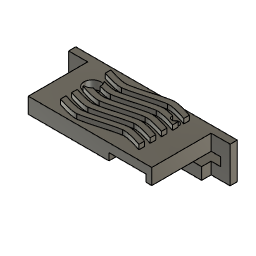
Enviro Module Cover Plate (Autodesk Fusion 360 design; units mm, degrees)
Autodesk Fusion 360 part; units mm, degrees
sketch "Sketch1" plane through (0, 0, 0) normal (0, 0, 1) x (1, 0, 0)
  line L0 (0, 0) -> (26, 0)
  line L1 (26, 0) -> (26, 16)
  line L2 (26, 16) -> (0, 16)
  line L3 (0, 16) -> (0, 0)
  dimension "d1" = 26
  dimension "d2" = 16
  constraint horizontal L0
  constraint vertical L1
  constraint horizontal L2
  constraint vertical L3
  constraint coincident L0.start L3.end
  measures "d1" horizontal distance of L0.start L0.end
  measures "d2" vertical distance of L0.start L2.end
extrude "Extrude1" add sketch "Sketch1" along normal blind 3.3
sketch "Sketch2" plane through (0, 0, 0) normal (0, 0, 1) x (1, 0, 0)
  line L0 (0, 16) -> (26, 16)
  line L1 (26, 16) -> (26, 14.5)
  line L2 (26, 14.5) -> (0, 14.5)
  line L3 (0, 14.5) -> (0, 16)
  point P0 (0, 16)
  dimension "d5" = 1.5
  constraint horizontal L0
  constraint vertical L1
  constraint horizontal L2
  constraint vertical L3
  constraint coincident P0 L0.start
  measures "d5" vertical distance of P0 L2.end
extrude "Extrude2" add sketch "Sketch2" against normal blind 1.8
sketch "Sketch3" plane through (0, 0, 0) normal (0, 0, -1) x (1, 0, 0)
  line L0 (0, -14.5) -> (26, -14.5)
  line L1 (26, -14.5) -> (26, 0)
  line L2 (26, 0) -> (0, 0)
  line L3 (0, 0) -> (0, -14.5)
  line L4 (0, -10) -> (2, -10)
  line L5 (2, -10) -> (2, -4.5)
  line L6 (2, -4.5) -> (17, -4.5)
  line L7 (17, -4.5) -> (17, 0)
  line L8 (17, 0) -> (24.8, 0)
  line L9 (24.8, 0) -> (24.8, -14.5)
  line L10 (0, -11.5) -> (2, -11.5)
  line L11 (2, -11.5) -> (2, -14.5)
  dimension "d8" = 1.2
  dimension "d9" = 14.5
  dimension "d10" = 10
  dimension "d11" = 2
  dimension "d12" = 3
  dimension "d13" = 1.5
  dimension "d14" = 9
  constraint perpendicular L3 L4
  constraint perpendicular L4 L5
  constraint perpendicular L5 L6
  constraint perpendicular L6 L7
  constraint perpendicular L5 L8
  constraint perpendicular L0 L9
  constraint coincident L0 L9.end
  constraint coincident L3 L4.start
  constraint coincident L3 L10.start
  constraint perpendicular L3 L10
  constraint coincident L0 L11.end
  constraint perpendicular L0 L11
  constraint collinear L5 L11
  measures "d8" distance of L1 L9
  measures "d9" distance of L8 L9.end
  measures "d10" distance of L0 L6
  measures "d11" distance of L3 L11
  measures "d12" distance of L0 L10
  measures "d13" distance of L4 L10
  measures "d14" distance of L1 L7
extrude "Extrude3" cut sketch "Sketch3" against normal blind 1.5 contours L0 L2 L3 L4 L5 L6 L7 L8 L9 L10 L11
sketch "Sketch4" plane through (0, 0, -1.8) normal (0, 0, -1) x (1, 0, 0)
  line L0 (26, -14.5) -> (0, -14.5)
  line L1 (0, -14.5) -> (0, -16)
  line L2 (0, -16) -> (26, -16)
  line L3 (26, -16) -> (26, -14.5)
  line L4 (0, -16) -> (26, -16)
  line L5 (26, -16) -> (26, -10.5)
  line L6 (26, -10.5) -> (0, -10.5)
  line L7 (0, -10.5) -> (0, -16)
  line L8 (26, 0) -> (26, -16)
  dimension "d30" = 5.5
  constraint horizontal L4
  constraint vertical L5
  constraint horizontal L6
  constraint vertical L7
  constraint coincident L5.end L8
  constraint coincident L1.end L2.start
  measures "d30" distance of L4 L6
extrude "Extrude4" add sketch "Sketch4" along normal blind 2.5
sketch "Sketch5" plane through (0, 0, 3.3) normal (0, 0, 1) x (-1, 0, 0)
  line L0 (0, -16) -> (0, 0)
  line L1 (0, 0) -> (-26, 0)
  line L2 (-26, 0) -> (-26, -16)
  line L3 (-26, -16) -> (0, -16)
  circle A0 centre (-5, -8.5) radius 1.75
  circle A1 centre (-20.5, -10.5) radius 0.75
  line L4 (-24.8, -14.5) -> (-2, -14.5)
  dimension "d20" = 3.5
  dimension "d21" = 1.5
  dimension "d22" = 5
  dimension "d23" = 20.5
  dimension "d24" = 6
  dimension "d25" = 4
  measures "d20" diameter of A0
  measures "d21" diameter of A1
  measures "d22" distance of L0 A0.centre
  measures "d23" distance of L0 A1.centre
  measures "d24" distance of A0.centre L4
  measures "d25" distance of A1.centre L4
extrude "Extrude5" cut sketch "Sketch5" against normal up to surface (1.8 mm away) contours A0 | A1
sketch "Sketch6" plane through (0, 0, 3.3) normal (0, 0, 1) x (-1, 0, 0)
  circle A0 centre (-20.5, -10.5) radius 0.75
  circle A1 centre (-5, -8.5) radius 1.75
  line L0 (0, -16) -> (0, 0)
  line L1 (0, 0) -> (-26, 0)
  line L2 (-26, 0) -> (-26, -16)
  line L3 (-26, -16) -> (0, -16)
  line L4 (0, -16) -> (4, -16)
  line L5 (4, -16) -> (4, -12.5)
  line L6 (4, -12.5) -> (0, -12.5)
  line L7 (0, -14.5) -> (-2, -14.5)
  line L8 (0, -14.5) -> (2, -12.5)
  line L9 (-13, -26.5) -> (-13, -5.5) construction
  line L10 (0, -16) -> (0, -12.5)
  line L11 (-26, -16) -> (-26, -12.5)
  line L12 (-26, -14.5) -> (-28, -12.5)
  line L13 (-30, -12.5) -> (-26, -12.5)
  line L14 (-30, -16) -> (-30, -12.5)
  line L15 (-26, -16) -> (-30, -16)
  dimension "d31" = 45
  dimension "d32" = 3.5
  dimension "d33" = 4
  constraint coincident L0.start L3.end
  constraint perpendicular L0 L4
  constraint perpendicular L3 L5
  constraint coincident L0 L6.end
  constraint perpendicular L0 L6
  constraint coincident L7.start L8.start
  constraint coincident L6 L8.end
  constraint perpendicular L3 L9
  constraint midpoint L3 L9
  constraint symmetric L0.start L9 L2.end
  constraint symmetric L4.end L9 L14.start
  constraint symmetric L5.end L9 L13.start
  constraint symmetric L6.end L9 L11.end
  constraint symmetric L7.start L9 L12.start
  constraint symmetric L8.end L9 L12.end
  measures "d31" angle of L0 L8
  measures "d32" distance of L4.end L5.end
  measures "d33" distance of L0.start L4.end
extrude "Extrude6" add sketch "Sketch6" against normal up to surface (7.6 mm away) contours L0 L4 L5 L6 L8 L10 | L0 L6 L8 L10 | L2 L11 L12 L13 L14 L15 | L2 L11 L12 L13
extrude "Extrude7" cut sketch "Sketch6" against normal up to surface (1.8 mm away) from surface at -3.3 contours L0 L6 L8 L10 | L2 L11 L12 L13
chamfer "Chamfer2" distance 2 angle 45 4 edges at (13, 16, 3.3) (-4, 16, -0.5) (30, 16, -0.5) (13, 16, -4.3)
sketch "Sketch7" plane through (0, 0, 3.3) normal (0, 0, 1) x (-1, 0, 0)
  line L0 (-30, -14) -> (4, -14)
  line L1 (4, -14) -> (4, -12.5)
  line L2 (4, -12.5) -> (0, -12.5)
  line L3 (0, -12.5) -> (0, 0)
  line L4 (0, 0) -> (-26, 0)
  line L5 (-26, 0) -> (-26, -12.5)
  line L6 (-26, -12.5) -> (-30, -12.5)
  line L7 (-30, -12.5) -> (-30, -14)
  circle A0 centre (-20.5, -10.5) radius 0.75
  circle A1 centre (-5, -8.5) radius 1.75
  spline S0 degree 2 poles (-17.0598, -3.9964) (-18.1405, -4.1471) (-21.4242, -3.0527) knots 0 0 0 1 1 1
  line L8 (-21.4242, -3.0527) -> (-21.4242, -1.8731)
  spline S1 degree 2 poles (-21.4242, -1.8731) (-18.1405, -2.9676) (-17.0598, -2.8168) knots 0 0 0 1 1 1
  spline S2 degree 3 poles (-17.0598, -2.8168) (-15.0764, -2.5401) (-11.2633, -1.1671) (-9.2746, -0.9295) knots 0 0 0 0 1 1 1 1
  spline S3 degree 2 poles (-9.2746, -0.9295) (-8.191, -0.8) (-4.9101, -1.8731) knots 0 0 0 1 1 1
  line L9 (-4.9101, -1.8731) -> (-4.9101, -3.0527)
  spline S4 degree 2 poles (-4.9101, -3.0527) (-8.191, -1.9795) (-9.2746, -2.1091) knots 0 0 0 1 1 1
  spline S5 degree 3 poles (-9.2746, -2.1091) (-11.2633, -2.3466) (-15.0764, -3.7197) (-17.0598, -3.9964) knots 0 0 0 0 1 1 1 1
  spline S6 degree 2 poles (-17.0598, -6.3539) (-18.1405, -6.5046) (-21.4242, -5.4102) knots 0 0 0 1 1 1
  line L10 (-21.4242, -5.4102) -> (-21.4242, -4.2306)
  spline S7 degree 2 poles (-21.4242, -4.2306) (-18.1405, -5.3251) (-17.0598, -5.1743) knots 0 0 0 1 1 1
  spline S8 degree 3 poles (-17.0598, -5.1743) (-15.0764, -4.8976) (-11.2633, -3.5246) (-9.2746, -3.287) knots 0 0 0 0 1 1 1 1
  spline S9 degree 2 poles (-9.2746, -3.287) (-8.191, -3.1575) (-4.9101, -4.2306) knots 0 0 0 1 1 1
  line L11 (-4.9101, -4.2306) -> (-4.9101, -5.4102)
  spline S10 degree 2 poles (-4.9101, -5.4102) (-8.191, -4.337) (-9.2746, -4.4666) knots 0 0 0 1 1 1
  spline S11 degree 3 poles (-9.2746, -4.4666) (-11.2633, -4.7041) (-15.0764, -6.0772) (-17.0598, -6.3539) knots 0 0 0 0 1 1 1 1
  spline S12 degree 2 poles (-17.0598, -8.713) (-18.1405, -8.8638) (-21.4242, -7.7694) knots 0 0 0 1 1 1
  line L12 (-21.4242, -7.7694) -> (-21.4242, -6.5898)
  spline S13 degree 2 poles (-21.4242, -6.5898) (-18.1405, -7.6842) (-17.0598, -7.5335) knots 0 0 0 1 1 1
  spline S14 degree 3 poles (-17.0598, -7.5335) (-15.0764, -7.2567) (-11.2633, -5.8835) (-9.2746, -5.6461) knots 0 0 0 0 1 1 1 1
  spline S15 degree 2 poles (-9.2746, -5.6461) (-8.191, -5.5166) (-4.9101, -6.5898) knots 0 0 0 1 1 1
  line L13 (-4.9101, -6.5898) -> (-4.9101, -7.7694)
  spline S16 degree 2 poles (-4.9101, -7.7694) (-8.191, -6.6962) (-9.2746, -6.8257) knots 0 0 0 1 1 1
  spline S17 degree 3 poles (-9.2746, -6.8257) (-11.2633, -7.0633) (-15.0764, -8.4363) (-17.0598, -8.713) knots 0 0 0 0 1 1 1 1
  spline S18 degree 2 poles (-17.0598, -11.0722) (-18.1405, -11.2229) (-21.4242, -10.1285) knots 0 0 0 1 1 1
  line L14 (-21.4242, -10.1285) -> (-21.4242, -8.949)
  spline S19 degree 2 poles (-21.4242, -8.949) (-18.1405, -10.0434) (-17.0598, -9.8926) knots 0 0 0 1 1 1
  spline S20 degree 3 poles (-17.0598, -9.8926) (-15.0764, -9.6159) (-11.2633, -8.2429) (-9.2746, -8.0053) knots 0 0 0 0 1 1 1 1
  spline S21 degree 2 poles (-9.2746, -8.0053) (-8.191, -7.8758) (-4.9101, -8.949) knots 0 0 0 1 1 1
  line L15 (-4.9101, -8.949) -> (-4.9101, -10.1285)
  spline S22 degree 2 poles (-4.9101, -10.1285) (-8.191, -9.0554) (-9.2746, -9.1849) knots 0 0 0 1 1 1
  spline S23 degree 3 poles (-9.2746, -9.1849) (-11.2633, -9.4224) (-15.0764, -10.7955) (-17.0598, -11.0722) knots 0 0 0 0 1 1 1 1
  spline S24 degree 2 poles (-17.0598, -13.4313) (-18.1405, -13.5821) (-21.4242, -12.4877) knots 0 0 0 1 1 1
  line L16 (-21.4242, -12.4877) -> (-21.4242, -11.3081)
  spline S25 degree 2 poles (-21.4242, -11.3081) (-18.1405, -12.4025) (-17.0598, -12.2518) knots 0 0 0 1 1 1
  spline S26 degree 3 poles (-17.0598, -12.2518) (-15.0764, -11.975) (-11.2633, -10.602) (-9.2746, -10.3644) knots 0 0 0 0 1 1 1 1
  spline S27 degree 2 poles (-9.2746, -10.3644) (-8.191, -10.2349) (-4.9101, -11.3081) knots 0 0 0 1 1 1
  line L17 (-4.9101, -11.3081) -> (-4.9101, -12.4877)
  spline S28 degree 2 poles (-4.9101, -12.4877) (-8.191, -11.4145) (-9.2746, -11.544) knots 0 0 0 1 1 1
  spline S29 degree 3 poles (-9.2746, -11.544) (-11.2633, -11.7816) (-15.0764, -13.1546) (-17.0598, -13.4313) knots 0 0 0 0 1 1 1 1
extrude "Extrude8" add sketch "Sketch7" along normal blind 1 contours A0 A1 S18 L14 S19 S20 S21 S22 S23 | A1 S12 L12 S13 S14 S15 L13 S16 S17 | S0 L8 S1 S2 S3 L9 S4 S5 | S6 L10 S7 S8 S9 L11 S10 S11 | S24 L16 S25 S26 S27 L17 S28 S29
equation "d2 = 14.5 mm + topThickness"
equation "d5 = topThickness"
equation "topThickness = 1.5 mm"
equation "d30 = 4 mm + topThickness"
equation "d32 = 2 mm + topThickness"
